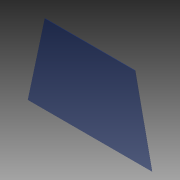
# Autodesk Inventor part: front window
Saved by Autodesk Inventor 2012 (Build 160160000, 160)
## iProperties
Created: 2011-12-02
Part Number: front window
Material: Polycarbonate, Clear
Document SubType Name: Modeling
Designer: Antonella
Mass: 189.206 g
Surface Area: 2007.51 cm^2
Volume: 157.671 cm^3
Density: 1.2 g/cm^3
Author: Antonella
Autodesk Inventor part; units mm, degrees
ref_plane "YZ Plane" through (0, 0, 0) normal (1, 0, 0) x (0, 1, 0)
ref_plane "XZ Plane" through (0, 0, 0) normal (0, 1, 0) x (-1, 0, 0)
ref_plane "XY Plane" through (0, 0, 0) normal (0, 0, 1) x (1, 0, 0)
sketch "Sketch1" plane through (0, 0, 0) normal (0, 0, 1) x (1, 0, 0)
  line L0 (-342.265, 0) -> (342.265, 0) projected
  line L1 (0, -62.23) -> (0, 373.38) projected
  line L2 (-177.8, 311.15) -> (177.8, 311.15)
  line L3 (177.8, 311.15) -> (244.475, 0)
  line L4 (244.475, 0) -> (-244.475, 0)
  line L5 (-244.475, 0) -> (-177.8, 311.15)
  point P0 (0, 0)
  point P1 (0, 311.15)
  dimension "d0" = 355.6
  dimension "d1" = 488.95
  dimension "d5" = 311.15
  constraints: 8 end point, 1 collinear, 1 equal length, 1 midpoint, 1 parallel, 1 perpendicular, 1 vertical alignment
  measures "d0" distance of L2.start L2.end
  measures "d1" distance of L3.end L4.end
  measures "d5" distance between parallel lines of L2 L0
extrude "Extrusion1" add sketch "Sketch1" along normal blind 1.5875
body "Solid1"
